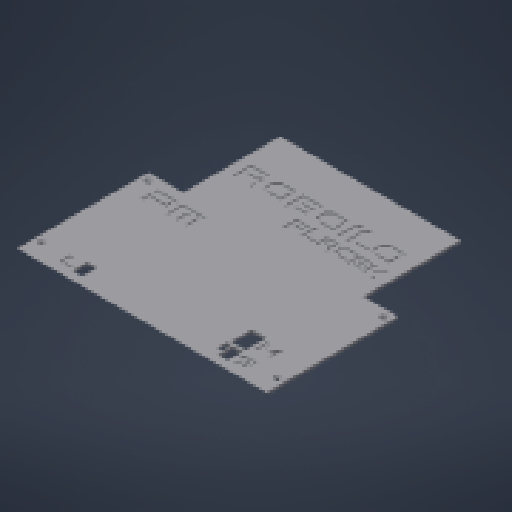
# Autodesk Inventor part: dach3
Saved by Autodesk Inventor 2023 (Build 270158000, 158)
## iProperties
Created: 2019-09-08
Part Number: dach3
Material: Generic
Document SubType Name: Modeling
Designer: Michal
Density: 1 g/cm^3
Appearance: Default
Author: Michal
Autodesk Inventor part; units mm, degrees
ref_plane "YZ Plane" through (0, 0, 0) normal (1, 0, 0) x (0, 1, 0)
ref_plane "XZ Plane" through (0, 0, 0) normal (0, 1, 0) x (-1, 0, 0)
ref_plane "XY Plane" through (0, 0, 0) normal (0, 0, 1) x (1, 0, 0)
sketch "Sketch1" plane through (0, 0, 0) normal (0, 1, 0) x (-1, 0, 0)
  line L0 (0, 0) -> (180, 0)
  line L1 (180, 0) -> (180, -95)
  line L2 (0, 0) -> (0, -95)
  line L3 (180, -95) -> (155, -95)
  line L4 (0, -95) -> (25, -95)
  line L5 (25, -95) -> (25, -165)
  line L6 (155, -95) -> (155, -165)
  line L7 (155, -165) -> (25, -165)
  dimension "d0" = 180
  dimension "d1" = 95
  dimension "d4" = 95
  dimension "d35" = 25
  dimension "d36" = 25
  constraints: 16 end point, 4 horizontal, 2 perpendicular, 2 vertical
  measures "d0" distance of L0.start L0.end
  measures "d1" distance of L0.end L1.end
  measures "d4" distance of L0.start L2.end
  measures "d35" distance of L1.end L3.end
  measures "d36" distance of L2.end L4.end
extrude "Extrusion1" add sketch "Sketch1" along normal blind 2
chamfer "Chamfer1" distance 2 angle 45 1 edges at (-90, 0, 0)
sketch "Sketch7" plane through (0, 2, 0) normal (0, 1, 0) x (1, 0, 0)
  line L0 (-155, 95) -> (-180, 95) projected
  line L1 (-180, 95) -> (-175, 95)
  line L2 (-175, 95) -> (-175, 90)
  line L3 (-175, 90) -> (-180, 90)
  line L4 (-180, 90) -> (-180, 95)
  line L5 (0, 95) -> (-25, 95) projected
  line L6 (0, 95) -> (-5, 95)
  line L7 (-5, 95) -> (-5, 90)
  line L8 (-5, 90) -> (0, 90)
  line L9 (0, 90) -> (0, 95)
  line L10 (-5, 90) -> (-5, 13)
  line L11 (-175, 90) -> (-175, 13)
  point P0 (0, 0)
  dimension "d80" = 5
  dimension "d81" = 5
  dimension "d82" = 5
  dimension "d83" = 77
  constraints: 20 end point, 4 parallel, 2 horizontal, 2 perpendicular, 2 vertical, 1 point on line
  measures "d80" distance of L2.end L3.end
  measures "d81" distance of L1.end L2.end
  measures "d82" distance of L8.end L7.end
  measures "d83" distance of L7.end L10.end
hole "Hole1" at (-175, 2, -90) at (-5, 2, -90) at (-5, 2, -13) at (-175, 2, -13) direction (0, -1, 0) diameter 2.4638 depth 8.7884 countersink diameter 5 countersink angle 75
sketch "Sketch8" plane through (0, 2, 0) normal (0, 1, 0) x (1, 0, 0)
  line L0 (0, 0) -> (0, 95) projected
  line L1 (-180, 95) -> (-180, 0) projected
  line L2 (-180, 0) -> (0, 0) projected
  line L3 (-180, 0) -> (-145, 0)
  line L4 (-180, 22.0001) -> (-180, 0)
  line L5 (-155, 95) -> (-180, 95) projected
  line L6 (-180, 95) -> (-180, 17)
  line L7 (-180, 17) -> (-146, 17)
  line L8 (-25, 165) -> (-155, 165) projected
  line L9 (-90, 165) -> (-90, 0)
  line L10 (-41, 17) -> (-34, 17)
  line L11 (-139, 17) -> (-146, 17)
  line L12 (-41, 17) -> (-41, 6)
  line L13 (-41, 6) -> (-34, 6)
  line L14 (-34, 6) -> (-34, 17)
  line L15 (-139, 17) -> (-139, 6)
  line L16 (-139, 6) -> (-146, 6)
  line L17 (-146, 6) -> (-146, 17)
  line L18 (-34, 17) -> (-34, 19)
  line L19 (-34, 19) -> (-44.5, 19)
  line L20 (-44.5, 19) -> (-44.5, 34)
  line L21 (-44.5, 34) -> (-34, 34)
  line L22 (-34, 34) -> (-34, 19)
  line L23 (-41, 17) -> (-42, 17)
  line L24 (-42, 17) -> (-42, 10)
  line L25 (-42, 10) -> (-45.5, 10)
  line L26 (-45.5, 10) -> (-45.5, 17)
  line L27 (-45.5, 17) -> (-42, 17)
  dimension "d266" = 78
  dimension "d267" = 34
  dimension "d275" = 11
  dimension "d276" = 7
  dimension "d277" = 11
  dimension "d278" = 7
  dimension "d290" = 2
  dimension "d291" = 10.5
  dimension "d292" = 15
  dimension "d297" = 1
  dimension "d298" = 7
  dimension "d299" = 3.5
  constraints: 46 end point, 10 perpendicular, 4 vertical, 3 horizontal, 3 point on line, 2 midpoint, 1 coincident, 1 parallel, 1 symmetric about line
  measures "d266" distance of L1.start L6.end
  measures "d267" distance of L6.end L7.end
  measures "d275" distance of L10.start L12.end
  measures "d276" distance of L12.end L13.end
  measures "d277" distance of L11.start L15.end
  measures "d278" distance of L15.end L16.end
  measures "d290" distance of L10.end L18.end
  measures "d291" distance of L18.end L19.end
  measures "d292" distance of L19.end L20.end
  measures "d297" distance of L10.start L23.end
  measures "d298" distance of L23.end L24.end
  measures "d299" distance of L24.end L25.end
extrude "Extrusion7" cut sketch "Sketch8" against normal blind 7
sketch "Sketch5" plane through (0, 2, 0) normal (0, 1, 0) x (1, 0, 0)
  line L0 (-154.7367, 165.2131) -> (-24.9468, 165.2131) construction
  line L1 (-24.9468, 165.2131) -> (-24.9468, 95.1481) construction
  line L2 (-24.9468, 95.1481) -> (-154.7367, 95.1481) construction
  line L3 (-154.7367, 95.1481) -> (-154.7367, 165.2131) construction
  line L4 (-180, 2) -> (-180, 95) projected
  line L5 (-166.0933, 87.2081) -> (-150.8913, 87.2081)
  line L6 (-150.8913, 87.2081) -> (-150.8913, 78.7451)
  line L7 (-166.0933, 87.2081) -> (-166.0933, 84.5691)
  line L8 (-166.0933, 84.5691) -> (-153.5243, 84.5691)
  line L9 (-153.5243, 84.5691) -> (-153.5243, 81.3771)
  line L10 (-153.5243, 81.3771) -> (-166.0933, 81.3771)
  line L11 (-166.0933, 81.3771) -> (-166.0933, 75.6831)
  line L12 (-166.0933, 75.6831) -> (-163.4573, 75.6831)
  line L13 (-163.4573, 75.6831) -> (-163.4573, 78.7451)
  line L14 (-163.4573, 78.7451) -> (-150.8913, 78.7451)
  line L15 (-150.8913, 87.2081) -> (-147.5843, 87.2081)
  line L16 (-147.5843, 87.2081) -> (-147.5843, 75.6831)
  line L17 (-147.5843, 75.6831) -> (-144.9503, 75.6831)
  line L18 (-144.9503, 75.6831) -> (-144.9503, 84.5691)
  line L19 (-144.9503, 84.5691) -> (-133.8883, 84.5691)
  line L20 (-133.8883, 84.5691) -> (-133.8883, 75.6831)
  line L21 (-133.8883, 75.6831) -> (-131.2543, 75.6831)
  line L22 (-131.2543, 75.6831) -> (-131.2543, 87.2081)
  line L23 (-131.2543, 87.2081) -> (-147.5843, 87.2081)
  line L24 (-144.9503, 84.5691) -> (-140.7343, 84.5691)
  line L25 (-133.8883, 84.5691) -> (-138.1043, 84.5691)
  line L26 (-138.1043, 84.5691) -> (-138.1043, 83.0161)
  line L27 (-138.1043, 83.0161) -> (-140.7343, 83.0161)
  line L28 (-140.7343, 83.0161) -> (-140.7343, 75.6831)
  line L29 (-140.7343, 75.6831) -> (-138.1043, 75.6831)
  line L30 (-138.1043, 75.6831) -> (-138.1043, 83.0161)
  line L31 (-97.4333, 120.7168) -> (-29.5125, 120.7168) construction
  line L32 (-29.5125, 120.7168) -> (-29.5125, 109.0375) construction
  line L33 (-29.5125, 109.0375) -> (-97.4333, 109.0375) construction
  line L34 (-97.4333, 109.0375) -> (-97.4333, 120.7168) construction
  line L35 (-156.6685, 15.8327) -> (-147.6087, 15.8327) construction
  line L36 (-147.6087, 15.8327) -> (-147.6087, 6.9134) construction
  line L37 (-147.6087, 6.9134) -> (-156.6685, 6.9134) construction
  line L38 (-156.6685, 6.9134) -> (-156.6685, 15.8327) construction
  line L39 (-31.5864, 15.3091) -> (-20.1078, 15.3091) construction
  line L40 (-20.1078, 15.3091) -> (-20.1078, 7.731) construction
  line L41 (-20.1078, 7.731) -> (-31.5864, 7.731) construction
  line L42 (-31.5864, 7.731) -> (-31.5864, 15.3091) construction
  line L43 (-31.0414, 31.5464) -> (-18.0167, 31.5464) construction
  line L44 (-18.0167, 31.5464) -> (-18.0167, 22.6564) construction
  line L45 (-18.0167, 22.6564) -> (-31.0414, 22.6564) construction
  line L46 (-31.0414, 22.6564) -> (-31.0414, 31.5464) construction
  line L47 (-131.1694, 121.4211) -> (-135.0949, 123.67)
  line L48 (-135.0949, 123.67) -> (-135.0949, 126.8525)
  line L49 (-135.0949, 126.8525) -> (-136.2896, 128.0171)
  line L50 (-136.2896, 128.0171) -> (-143.7891, 128.0171)
  line L51 (-143.7891, 128.0171) -> (-143.7891, 123.67)
  line L52 (-143.7891, 123.67) -> (-147.7146, 123.67)
  line L53 (-147.7146, 123.67) -> (-147.7146, 136.6611)
  line L54 (-147.7146, 136.6611) -> (-134.1311, 136.6611)
  line L55 (-134.1311, 136.6611) -> (-131.1694, 132.6754)
  line L56 (-131.1694, 132.6754) -> (-133.4183, 129.6535)
  line L57 (-133.4183, 129.6535) -> (-131.1694, 127.3946)
  line L58 (-131.1694, 127.3946) -> (-131.1694, 121.4211)
  line L59 (-135.2053, 132.4044) -> (-136.2494, 133.7697)
  line L60 (-136.2494, 133.7697) -> (-143.7891, 133.7697)
  line L61 (-143.7891, 133.7697) -> (-143.7891, 130.9687)
  line L62 (-143.7891, 130.9687) -> (-136.2595, 130.9687)
  line L63 (-136.2595, 130.9687) -> (-135.2053, 132.4044)
  line L64 (-112.1947, 126.6216) -> (-115.1464, 123.67)
  line L65 (-115.1464, 123.67) -> (-125.989, 123.67)
  line L66 (-125.989, 123.67) -> (-128.9407, 126.6216)
  line L67 (-128.9407, 126.6216) -> (-128.9407, 133.7095)
  line L68 (-128.9407, 133.7095) -> (-125.989, 136.6611)
  line L69 (-125.989, 136.6611) -> (-115.1464, 136.6611)
  line L70 (-115.1464, 136.6611) -> (-112.1947, 133.7095)
  line L71 (-112.1947, 133.7095) -> (-112.1947, 126.6216)
  line L72 (-116.1202, 126.5614) -> (-116.1202, 133.7697)
  line L73 (-116.1202, 133.7697) -> (-125.0152, 133.7697)
  line L74 (-125.0152, 133.7697) -> (-125.0152, 126.5614)
  line L75 (-125.0152, 126.5614) -> (-116.1202, 126.5614)
  line L76 (-93.3807, 127.6456) -> (-96.3323, 123.6499)
  line L77 (-96.3323, 123.6499) -> (-110.0965, 123.6499)
  line L78 (-110.0965, 123.6499) -> (-110.0965, 136.6611)
  line L79 (-110.0965, 136.6611) -> (-96.3323, 136.6611)
  line L80 (-96.3323, 136.6611) -> (-93.3807, 132.6654)
  line L81 (-93.3807, 132.6654) -> (-95.2279, 130.1555)
  line L82 (-95.2279, 130.1555) -> (-93.3807, 127.6456)
  line L83 (-97.6776, 127.6456) -> (-98.6313, 128.8303)
  line L84 (-98.6313, 128.8303) -> (-106.171, 128.8303)
  line L85 (-106.171, 128.8303) -> (-106.171, 126.5614)
  line L86 (-106.171, 126.5614) -> (-98.6313, 126.5614)
  line L87 (-98.6313, 126.5614) -> (-97.6776, 127.6456)
  line L88 (-97.6776, 132.6654) -> (-98.6313, 133.7497)
  line L89 (-98.6313, 133.7497) -> (-106.171, 133.7497)
  line L90 (-106.171, 133.7497) -> (-106.171, 131.4807)
  line L91 (-106.171, 131.4807) -> (-98.6313, 131.4807)
  line L92 (-98.6313, 131.4807) -> (-97.6776, 132.6654)
  line L93 (-74.5766, 126.6216) -> (-77.5283, 123.67)
  line L94 (-77.5283, 123.67) -> (-88.3709, 123.67)
  line L95 (-88.3709, 123.67) -> (-91.3226, 126.6216)
  line L96 (-91.3226, 126.6216) -> (-91.3226, 133.7095)
  line L97 (-91.3226, 133.7095) -> (-88.3709, 136.6611)
  line L98 (-88.3709, 136.6611) -> (-77.5283, 136.6611)
  line L99 (-77.5283, 136.6611) -> (-74.5766, 133.7095)
  line L100 (-74.5766, 133.7095) -> (-74.5766, 126.6216)
  line L101 (-78.5021, 126.5614) -> (-78.5021, 133.7697)
  line L102 (-78.5021, 133.7697) -> (-87.3971, 133.7697)
  line L103 (-87.3971, 133.7697) -> (-87.3971, 126.5614)
  line L104 (-87.3971, 126.5614) -> (-78.5021, 126.5614)
  line L105 (-68.5529, 123.6499) -> (-72.4784, 123.67)
  line L106 (-72.4784, 123.67) -> (-72.4784, 136.6712)
  line L107 (-72.4784, 136.6712) -> (-68.5529, 138.9401)
  line L108 (-68.5529, 138.9401) -> (-68.5529, 123.6499)
  line L109 (-51.2347, 126.5614) -> (-54.1462, 123.6499)
  line L110 (-54.1462, 123.6499) -> (-66.3241, 123.6499)
  line L111 (-66.3241, 123.6499) -> (-66.3241, 136.6712)
  line L112 (-66.3241, 136.6712) -> (-62.3987, 138.9401)
  line L113 (-62.3987, 138.9401) -> (-62.3987, 126.5614)
  line L114 (-62.3987, 126.5614) -> (-51.2347, 126.5614)
  line L115 (-34.0471, 126.6216) -> (-36.9987, 123.67)
  line L116 (-36.9987, 123.67) -> (-47.8414, 123.67)
  line L117 (-47.8414, 123.67) -> (-50.793, 126.6216)
  line L118 (-50.793, 126.6216) -> (-50.793, 133.7095)
  line L119 (-50.793, 133.7095) -> (-47.8414, 136.6611)
  line L120 (-47.8414, 136.6611) -> (-36.9987, 136.6611)
  line L121 (-36.9987, 136.6611) -> (-34.0471, 133.7095)
  line L122 (-34.0471, 133.7095) -> (-34.0471, 126.6216)
  line L123 (-37.9725, 126.5614) -> (-37.9725, 133.7697)
  line L124 (-37.9725, 133.7697) -> (-46.8675, 133.7697)
  line L125 (-46.8675, 133.7697) -> (-46.8675, 126.5614)
  line L126 (-46.8675, 126.5614) -> (-37.9725, 126.5614)
  line L127 (-86.3965, 116.5403) -> (-88.6922, 113.4348)
  line L128 (-88.6922, 113.4348) -> (-94.8096, 113.4348)
  line L129 (-94.8096, 113.4348) -> (-94.8096, 110.5367)
  line L130 (-94.8096, 110.5367) -> (-97.4266, 109.0375)
  line L131 (-97.4266, 109.0375) -> (-97.4266, 119.1975)
  line L132 (-97.4266, 119.1975) -> (-88.3709, 119.1975)
  line L133 (-88.3709, 119.1975) -> (-86.3965, 116.5403)
  line L134 (-89.0938, 116.3596) -> (-89.7831, 117.2699)
  line L135 (-89.7831, 117.2699) -> (-94.8096, 117.2699)
  line L136 (-94.8096, 117.2699) -> (-94.8096, 115.4025)
  line L137 (-94.8096, 115.4025) -> (-89.7831, 115.4025)
  line L138 (-89.7831, 115.4025) -> (-89.0938, 116.3596)
  line L139 (-75.4802, 112.4643) -> (-77.4211, 110.5233)
  line L140 (-77.4211, 110.5233) -> (-85.5398, 110.5233)
  line L141 (-85.5398, 110.5233) -> (-85.5398, 119.2042)
  line L142 (-85.5398, 119.2042) -> (-82.9228, 120.7168)
  line L143 (-82.9228, 120.7168) -> (-82.9228, 112.4643)
  line L144 (-82.9228, 112.4643) -> (-75.4802, 112.4643)
  line L145 (-64.6709, 109.0375) -> (-67.3013, 110.5233)
  line L146 (-67.3013, 110.5233) -> (-67.3013, 113.0198)
  line L147 (-67.3013, 113.0198) -> (-72.5687, 113.0198)
  line L148 (-72.5687, 113.0198) -> (-72.5687, 110.5233)
  line L149 (-72.5687, 110.5233) -> (-75.1857, 110.5367)
  line L150 (-75.1857, 110.5367) -> (-75.1857, 117.2565)
  line L151 (-75.1857, 117.2565) -> (-73.2179, 119.1975)
  line L152 (-73.2179, 119.1975) -> (-66.6387, 119.1975)
  line L153 (-66.6387, 119.1975) -> (-64.6709, 117.2565)
  line L154 (-64.6709, 117.2565) -> (-64.6709, 109.0375)
  line L155 (-67.3013, 114.934) -> (-67.3013, 117.2565)
  line L156 (-67.3013, 117.2565) -> (-72.5687, 117.2565)
  line L157 (-72.5687, 117.2565) -> (-72.5687, 114.934)
  line L158 (-72.5687, 114.934) -> (-67.3013, 114.934)
  line L159 (-52.7908, 119.1975) -> (-54.7184, 117.2565)
  line L160 (-54.7184, 117.2565) -> (-60.5414, 117.2565)
  line L161 (-60.5414, 117.2565) -> (-60.5414, 112.4643)
  line L162 (-60.5414, 112.4643) -> (-53.0987, 112.4643)
  line L163 (-53.0987, 112.4643) -> (-55.0397, 110.5233)
  line L164 (-55.0397, 110.5233) -> (-61.1906, 110.5233)
  line L165 (-61.1906, 110.5233) -> (-63.1583, 112.4643)
  line L166 (-63.1583, 112.4643) -> (-63.1583, 117.2163)
  line L167 (-63.1583, 117.2163) -> (-61.1906, 119.1975)
  line L168 (-61.1906, 119.1975) -> (-52.7908, 119.1975)
  line L169 (-41.8344, 119.1975) -> (-43.762, 117.2565)
  line L170 (-43.762, 117.2565) -> (-49.5849, 117.2565)
  line L171 (-49.5849, 117.2565) -> (-49.5849, 115.7439)
  line L172 (-49.5849, 115.7439) -> (-43.0994, 115.7439)
  line L173 (-43.0994, 115.7439) -> (-44.8663, 113.9769)
  line L174 (-44.8663, 113.9769) -> (-49.5849, 113.9769)
  line L175 (-49.5849, 113.9769) -> (-49.5849, 112.4643)
  line L176 (-49.5849, 112.4643) -> (-42.1423, 112.4643)
  line L177 (-42.1423, 112.4643) -> (-44.0832, 110.5233)
  line L178 (-44.0832, 110.5233) -> (-52.2019, 110.5233)
  line L179 (-52.2019, 110.5233) -> (-52.2019, 119.1975)
  line L180 (-52.2019, 119.1975) -> (-41.8344, 119.1975)
  line L181 (-30.7507, 119.1975) -> (-34.0504, 116.0451)
  line L182 (-34.0504, 116.0451) -> (-31.0251, 113.0198)
  line L183 (-31.0251, 113.0198) -> (-31.0251, 110.5233)
  line L184 (-31.0251, 110.5233) -> (-33.6421, 109.0375)
  line L185 (-33.6421, 109.0375) -> (-33.6421, 112.6383)
  line L186 (-33.6421, 112.6383) -> (-35.5764, 114.5726)
  line L187 (-35.5764, 114.5726) -> (-38.3607, 111.9556)
  line L188 (-38.3607, 111.9556) -> (-38.3607, 110.5233)
  line L189 (-38.3607, 110.5233) -> (-40.9777, 110.5367)
  line L190 (-40.9777, 110.5367) -> (-40.9777, 119.1975)
  line L191 (-40.9777, 119.1975) -> (-38.3607, 119.1975)
  line L192 (-38.3607, 119.1975) -> (-38.3607, 114.9474)
  line L193 (-38.3607, 114.9474) -> (-33.8429, 119.1975)
  line L194 (-33.8429, 119.1975) -> (-30.7507, 119.1975)
  line L195 (-147.8605, 8.6118) -> (-149.5589, 6.9134)
  line L196 (-149.5589, 6.9134) -> (-156.6627, 6.9134)
  line L197 (-156.6627, 6.9134) -> (-156.6627, 14.5092)
  line L198 (-156.6627, 14.5092) -> (-154.3728, 15.8327)
  line L199 (-154.3728, 15.8327) -> (-154.3728, 8.6118)
  line L200 (-154.3728, 8.6118) -> (-147.8605, 8.6118)
  line L201 (-21.0566, 10.0618) -> (-22.7784, 7.731)
  line L202 (-22.7784, 7.731) -> (-31.5805, 7.731)
  line L203 (-31.5805, 7.731) -> (-29.8939, 9.4176)
  line L204 (-29.8939, 9.4176) -> (-24.1195, 9.4176)
  line L205 (-24.1195, 9.4176) -> (-23.5807, 10.0618)
  line L206 (-23.5807, 10.0618) -> (-24.1136, 10.7412)
  line L207 (-24.1136, 10.7412) -> (-29.9056, 10.7412)
  line L208 (-29.9056, 10.7412) -> (-31.5805, 12.9783)
  line L209 (-31.5805, 12.9783) -> (-29.8587, 15.3091)
  line L210 (-29.8587, 15.3091) -> (-21.0566, 15.3091)
  line L211 (-21.0566, 15.3091) -> (-22.7549, 13.6225)
  line L212 (-22.7549, 13.6225) -> (-28.5176, 13.6225)
  line L213 (-28.5176, 13.6225) -> (-29.074, 12.9783)
  line L214 (-29.074, 12.9783) -> (-28.5176, 12.299)
  line L215 (-28.5176, 12.299) -> (-22.7257, 12.299)
  line L216 (-22.7257, 12.299) -> (-21.0566, 10.0618)
  line L217 (-19.2993, 23.9683) -> (-21.5891, 23.9683)
  line L218 (-21.5891, 23.9683) -> (-21.5891, 28.8173)
  line L219 (-21.5891, 28.8173) -> (-24.4353, 24.9111)
  line L220 (-24.4353, 24.9111) -> (-25.917, 24.9111)
  line L221 (-25.917, 24.9111) -> (-28.7456, 28.8173)
  line L222 (-28.7456, 28.8173) -> (-28.7456, 23.9683)
  line L223 (-28.7456, 23.9683) -> (-31.0355, 22.6564)
  line L224 (-31.0355, 22.6564) -> (-31.0355, 31.5464)
  line L225 (-31.0355, 31.5464) -> (-28.447, 31.5464)
  line L226 (-28.447, 31.5464) -> (-25.1674, 27.037)
  line L227 (-25.1674, 27.037) -> (-21.8995, 31.5464)
  line L228 (-21.8995, 31.5464) -> (-19.2993, 31.5464)
  line L229 (-19.2993, 31.5464) -> (-19.2993, 23.9683)
  point P0 (0, 0)
  dimension "d166" = 15.202
  dimension "d167" = 8.463
  dimension "d168" = 2.639
  dimension "d169" = 12.569
  dimension "d170" = 3.192
  dimension "d171" = 5.694
  dimension "d172" = 2.636
  dimension "d173" = 3.307
  dimension "d174" = 2.634
  dimension "d175" = 8.886
  dimension "d176" = 11.062
  dimension "d177" = 2.634
  dimension "d178" = 4.216
  dimension "d179" = 4.216
  dimension "d180" = 1.553
  constraints: 52 end point, 15 perpendicular, 7 point on line, 3 horizontal, 3 parallel, 1 vertical, 10 other
  measures "d166" distance of L5.start L5.end
  measures "d167" distance of L5.end L6.end
  measures "d168" distance of L5.start L7.end
  measures "d169" distance of L7.end L8.end
  measures "d170" distance of L8.end L9.end
  measures "d171" distance of L10.end L11.end
  measures "d172" distance of L11.end L12.end
  measures "d173" distance of L5.end L15.end
  measures "d174" distance of L16.end L17.end
  measures "d175" distance of L17.end L18.end
  measures "d176" distance of L18.end L19.end
  measures "d177" distance of L20.end L21.end
  measures "d178" distance of L18.end L24.end
  measures "d179" distance of L19.end L25.end
  measures "d180" distance of L25.end L26.end
extrude "Extrusion6" cut sketch "Sketch5" against normal blind 1
body "Solid1"
